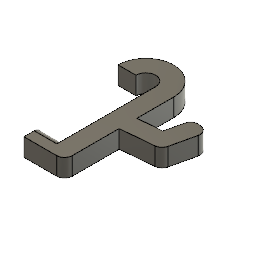
Short Lay Hook (Autodesk Fusion 360 design; units mm, degrees)
Autodesk Fusion 360 part; units mm, degrees
sketch "Sketch1" plane through (0, 0, 0) normal (0, 1, 0) x (1, 0, 0)
  circle A0 centre (0, 0) radius 7.2
  circle A1 centre (0, 0) radius 2.55
  line L0 (7.2, 0) -> (2.55, 0)
  line L1 (2.55, 0) -> (2.55, -28.2)
  line L2 (2.55, -28.2) -> (7.2, -28.2)
  line L3 (7.2, -28.2) -> (7.2, 0)
  line L4 (7.2, -28.2) -> (-3.3, -28.2)
  line L5 (-3.3, -28.2) -> (-3.3, -23.55)
  line L6 (-3.3, -23.55) -> (7.2, -23.55)
  line L7 (7.2, -23.55) -> (7.2, -28.2)
  line L8 (2.55, 0) -> (-7.2, 0)
  line L9 (7.2, -4.2775) -> (7.2, -1.15)
  line L10 (7.2, -14.1) -> (17.1595, -13.2006)
  line L11 (17.1595, -13.2006) -> (16.7494, -8.6591)
  line L12 (16.7494, -8.6591) -> (6.7899, -9.5585)
  line L13 (6.7899, -9.5585) -> (7.2, -14.1)
  line L14 (17.1595, -13.2006) -> (12.6262, -12.1654)
  line L15 (12.6262, -12.1654) -> (14.8525, -2.4164)
  line L16 (14.8525, -2.4164) -> (19.3858, -3.4516)
  line L17 (19.3858, -3.4516) -> (17.1595, -13.2006)
  dimension "d1" = 14.4
  dimension "d2" = 5.1
  dimension "d3" = 4.65
  dimension "d4" = 28.2
  dimension "d5" = 10.5
  dimension "d6" = 4.65
  dimension "d16" = 10
  dimension "d17" = 4.56
  dimension "d18" = 4.65
  dimension "d19" = 10
  constraint coincident A0.centre A1.centre
  constraint concentric A0 A1
  constraint horizontal L0
  constraint vertical L1
  constraint horizontal L2
  constraint vertical L3
  constraint coincident A0 L0.start
  constraint coincident A1 L0.end
  constraint horizontal L4
  constraint vertical L5
  constraint horizontal L6
  constraint vertical L7
  constraint coincident A0 L8.end
  constraint perpendicular L1 L8
  constraint vertical L9
  constraint coincident L3 L9.end
  constraint perpendicular L10 L11
  constraint parallel L10 L12
  constraint parallel L11 L13
  constraint coincident L3 L10.start
  constraint perpendicular L14 L15
  constraint parallel L14 L16
  constraint parallel L15 L17
  constraint midpoint L3 L10.start
  measures "d1" diameter of A0
  measures "d2" diameter of A1
  measures "d3" horizontal distance of L1.end L2.end
  measures "d4" vertical distance of L0.start L2.end
  measures "d5" distance of L2.end L4.end
  measures "d6" distance of L2.end L6.end
  measures "d16" distance of L10.start L10.end
  measures "d17" distance of L10.start L12.end
  measures "d18" distance of L10.end L14.end
  measures "d19" distance of L10.end L16.end
extrude "Extrude1" add sketch "Sketch1" along normal blind 4.65 contours A0 A1 L0 L8 | A0 L1 L3 L6 L9 L12 L13 | A0 L0 L1 | L1 L2 L3 L4 L6 L7 | L1 L4 L5 L6 | L3 L10 L12 L14 L15 | L3 L12 L13 | L11 L12 L15 L16 L17 | L11 L12 L14 L15
fillet "Fillet1" radius 2 3 edges at (14.8525, 2.325, 2.4164) (19.3858, 2.325, 3.4516) (17.1595, 2.325, 13.2006)
fillet "Fillet2" radius 2 1 edges at (7.2, 2.325, 28.2)
fillet "Fillet3" radius 2 2 edges at (-0.375, 4.65, 23.55) (-0.375, 0, 23.55)
